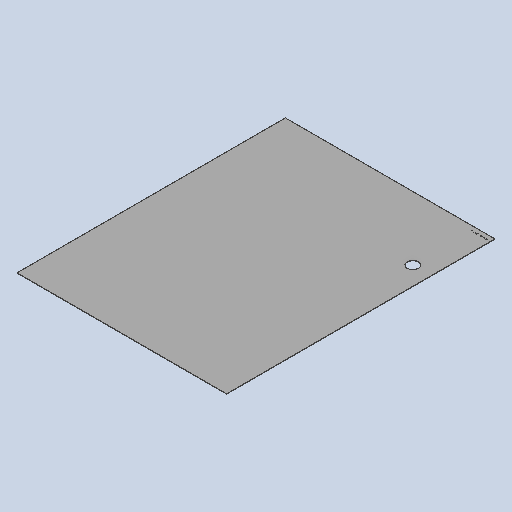
# Autodesk Inventor part: BSH 051 back 1
Saved by Autodesk Inventor 2025 (Build 290162010, 162A)
## iProperties
Created: 2024-07-23
Part Number: BSH 051 back 1
Material: 09g2s
Document SubType Name: Sheet Metal
Designer: pokla
Mass: 65930 g
Surface Area: 56201.5 cm^2
Volume: 8398.72 cm^3
Density: 7.85 g/cm^3
Sheet Metal Rule: AISI304 3mm Die 32
Sheet Metal Width: 1480,000 mm
Sheet Metal Length: 1895,000 mm
Sheet Metal Area: 2804600,000 mm^2
Appearance: Default
Flat Pattern Width: 148 cm
Flat Pattern Length: 189.5 cm
Flat Pattern Area: 28046 cm^2
Author: admin
Autodesk Inventor part; units mm, degrees
ref_plane "YZ Plane" through (0, 0, 0) normal (1, 0, 0) x (0, 1, 0)
ref_plane "XZ Plane" through (0, 0, 0) normal (0, 1, 0) x (-1, 0, 0)
ref_plane "XY Plane" through (0, 0, 0) normal (0, 0, 1) x (1, 0, 0)
sketch "Sketch6" plane through (0, 0, 0) normal (0, 0, 1) x (1, 0, 0)
  line L0 (740, 947.5) -> (-740, 947.5)
  line L1 (-740, 947.5) -> (-740, -947.5)
  line L2 (-740, -947.5) -> (740, -947.5)
  line L3 (740, -947.5) -> (740, 947.5)
  line L4 (740, 947.5) -> (-740, -947.5) construction
  line L5 (-740, 947.5) -> (740, -947.5) construction
  point P0 (0, 0)
  dimension "d40" = 1480
  dimension "d41" = 1895
  measures "d40" distance of L2.end L1.end
  measures "d41" distance of L1.end L0.end
extrude "Plate5" add sketch "Sketch6" along normal blind 3
sketch "Sketch7" plane through (0, 0, 0) normal (0, 0, -1) x (-1, 0, 0)
  line L0 (-715, 922.5) -> (-515, 922.5) construction
  line L1 (-515, 922.5) -> (-515, 907.5) construction
  line L2 (-515, 907.5) -> (-715, 907.5) construction
  line L3 (-715, 907.5) -> (-715, 922.5) construction
  line L4 (-740, 947.5) -> (740, 947.5) projected
  line L5 (-740, -947.5) -> (-740, 947.5) projected
  point P0 (0, 0)
  dimension "d43" = 200
  dimension "d44" = 15
  dimension "d45" = 25
  dimension "d46" = 25
  constraints: 2 parallel, 2 other
  measures "d43" distance of L3.end L0.end
  measures "d44" distance between parallel lines of L0 L2
  measures "d45" distance between parallel lines of L4 L0
  measures "d46" distance between parallel lines of L5 L3
mark "Mark1"
sketch "Sketch8" plane through (740, 947.5, 0) normal (0, 0, -1) x (-1, 0, 0)
  circle A0 centre (130, -450) radius 40
  line L0 (1480, 0) -> (1480, -1895) projected
  line L1 (0, 0) -> (1480, 0) projected
  point P0 (740, -947.5)
  dimension "d47" = 80
  dimension "d48" = 1350
  dimension "d49" = 450
  constraints: 1 centre point
  measures "d47" diameter of A0
  measures "d48" distance from line of L0 A0.centre
  measures "d49" distance from line of L1 A0.centre
extrude "Extrusion3" cut sketch "Sketch8" against normal up to surface (3 mm away)
equation "\"d42\" = Thickness"
equation "\"BendReliefWidth\" = Thickness"
equation "\"BendReliefDepth\" = 0.5 * Thickness"
equation "\"CornerReliefSize\" = 4 * Thickness"
equation "\"MinimumRemnant\" = 2 * Thickness"
equation "\"TransitionRadius\" = BendRadius"
equation "\"JacobiRadiusSize\" = BendRadius"
equation "\"GapSize\" = Thickness"
equation "\"Thickness\" = 3"
equation "\"BendRadius\" = 5"
body "Solid4"
